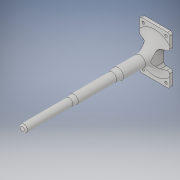
# Autodesk Inventor part: TapaInferiorConPata-v2
Saved by Autodesk Inventor 2019 (Build 230136000, 136)
## iProperties
Created: 2019-03-04
Part Number: TapaInferiorConPata-v2
Material: Generic
Document SubType Name: Modeling
Designer: Kenny
Density: 1 g/cm^3
Appearance: Default
Author: Kenny
Autodesk Inventor part; units mm, degrees
ref_plane "YZ Plane" through (0, 0, 0) normal (1, 0, 0) x (0, 1, 0)
ref_plane "XZ Plane" through (0, 0, 0) normal (0, 1, 0) x (-1, 0, 0)
ref_plane "XY Plane" through (0, 0, 0) normal (0, 0, 1) x (1, 0, 0)
sketch "Sketch1" plane through (0, 0, 0) normal (0, 0, 1) x (1, 0, 0)
  line L0 (41, 0) -> (41, 65.3) construction
  line L1 (0, 65.3) -> (0, 0) construction
  line L2 (41, 0) -> (41, 21)
  line L3 (0, 21) -> (0, 0)
  line L4 (41, 65.3) -> (41, 44.3)
  line L5 (0, 44.3) -> (0, 65.3)
  line L6 (29, 44.3) -> (29, 21)
  line L7 (12, 21) -> (12, 44.3)
  line L8 (41, 44.3) -> (29, 44.3)
  line L9 (12, 44.3) -> (0, 44.3)
  line L10 (41, 21) -> (29, 21)
  line L11 (12, 21) -> (0, 21)
  line L12 (41, 65.3) -> (30.5, 65.3) construction
  line L13 (10.5, 65.3) -> (0, 65.3) construction
  line L14 (0, 65.3) -> (10.5, 65.3)
  line L15 (30.5, 65.3) -> (41, 65.3)
  line L16 (0, 0) -> (10.5, 0) construction
  line L17 (30.5, 0) -> (41, 0) construction
  line L18 (0, 0) -> (10.5, 0)
  line L19 (30.5, 0) -> (41, 0)
  line L20 (10.5, 65.3) -> (30.5, 65.3)
  line L21 (10.5, 0) -> (30.5, 0)
  point P0 (5, 60.3)
  point P1 (36, 60.3)
  point P2 (5, 5)
  point P3 (36, 5)
  dimension "d0" = 41
  dimension "d1" = 65.3
  dimension "d2" = 21
  dimension "d3" = 21
  dimension "d4" = 12
  dimension "d9" = 5
  dimension "d11" = 5
  dimension "d12" = 41
  dimension "d13" = 41
  dimension "d14" = 12
  dimension "d19" = 5
  dimension "d20" = 5
  constraints: 44 end point, 17 parallel, 6 horizontal, 6 perpendicular, 2 horizontal alignment, 2 vertical alignment
  measures "d0" distance of L1.start L0.end
  measures "d1" distance of L0.end L0.start
  measures "d2" distance of L2.end L2.start
  measures "d3" distance of L4.start L4.end
  measures "d4" distance between parallel lines of L0 L6
  measures "d9" distance from line of L1 point (5, 60.3)
  measures "d11" distance from line of L0 point (36, 60.3)
  measures "d12" distance between parallel lines of L1 L2
  measures "d13" distance between parallel lines of L1 L4
  measures "d14" distance between parallel lines of L3 L7
  measures "d19" distance from line of L13 point (5, 60.3)
  measures "d20" distance from line of L16 point (5, 5)
extrude "Extrusion3" add sketch "Sketch1" along normal blind 4
sketch "Sketch5" plane through (0, 0, 0) normal (0, 0, 1) x (1, 0, 0)
  line L0 (41, 0) -> (41, 65.3) construction
  line L1 (0, 65.3) -> (0, 0) construction
  line L2 (41, 0) -> (41, 21)
  line L3 (0, 21) -> (0, 0)
  line L4 (41, 65.3) -> (41, 44.3)
  line L5 (0, 44.3) -> (0, 65.3)
  line L6 (29, 44.3) -> (29, 21)
  line L7 (12, 21) -> (12, 44.3)
  line L8 (41, 44.3) -> (29, 44.3)
  line L9 (12, 44.3) -> (0, 44.3)
  line L10 (41, 21) -> (29, 21)
  line L11 (12, 21) -> (0, 21)
  line L12 (30.5, 65.3) -> (30.5, 55.3)
  line L13 (30.5, 55.3) -> (10.5, 55.3)
  line L14 (10.5, 55.3) -> (10.5, 65.3)
  line L15 (41, 65.3) -> (30.5, 65.3) construction
  line L16 (10.5, 65.3) -> (0, 65.3) construction
  line L17 (0, 65.3) -> (10.5, 65.3)
  line L18 (30.5, 65.3) -> (41, 65.3)
  line L19 (10.5, 0) -> (10.5, 10)
  line L20 (10.5, 10) -> (30.5, 10)
  line L21 (30.5, 10) -> (30.5, 0)
  line L22 (0, 0) -> (10.5, 0) construction
  line L23 (30.5, 0) -> (41, 0) construction
  line L24 (0, 0) -> (10.5, 0)
  line L25 (30.5, 0) -> (41, 0)
  point P0 (5, 60.3)
  point P1 (36, 60.3)
  point P2 (5, 5)
  point P3 (36, 5)
  dimension "d53" = 41
  dimension "d54" = 65.3
  dimension "d55" = 21
  dimension "d56" = 21
  dimension "d57" = 12
  dimension "d58" = 5
  dimension "d59" = 5
  dimension "d60" = 41
  dimension "d61" = 41
  dimension "d62" = 12
  dimension "d63" = 10.5
  dimension "d64" = 10.5
  dimension "d65" = 5
  dimension "d66" = 5
  constraints: 52 end point, 18 parallel, 6 horizontal, 6 perpendicular, 2 horizontal alignment, 2 vertical alignment
  measures "d53" distance of L1.start L0.end
  measures "d54" distance of L0.end L0.start
  measures "d55" distance of L2.end L2.start
  measures "d56" distance of L4.start L4.end
  measures "d57" distance between parallel lines of L0 L6
  measures "d58" distance from line of L1 point (5, 60.3)
  measures "d59" distance from line of L0 point (36, 60.3)
  measures "d60" distance between parallel lines of L1 L2
  measures "d61" distance between parallel lines of L1 L4
  measures "d62" distance between parallel lines of L3 L7
  measures "d63" distance between parallel lines of L5 L14
  measures "d64" distance between parallel lines of L0 L12
  measures "d65" distance from line of L16 point (5, 60.3)
  measures "d66" distance from line of L22 point (5, 5)
hole "Hole2" at (5, 60.3, 0) at (36, 60.3, 0) at (5, 5, 0) at (36, 5, 0) direction (0, 0, 1) diameter 3.6 end through all
fillet "Fillet2" radius 3 12 edges at (0, 65.3, 2) (41, 65.3, 2) (41, 44.3, 2) (29, 44.3, 2) (29, 21, 2) (41, 21, 2) (41, 0, 2) (0, 0, 2) (0, 44.3, 2) (12, 44.3, 2) (12, 21, 2) (0, 21, 2)
sketch "Sketch6" plane through (0, 0, 4) normal (0, 0, 1) x (1, 0, 0)
  line L0 (12, 21) -> (12, 44.3) projected
  line L1 (29, 44.3) -> (29, 21) projected
  circle A0 centre (20.5, 32.65) radius 7.5
  line L2 (41, 65.3) -> (0, 65.3) projected
  point P0 (0, 0)
  dimension "d76" = 15
  dimension "d79" = 8.5
  dimension "d80" = 32.65
  constraints: 1 centre point
  measures "d76" diameter of A0
  measures "d79" distance from line of L1 A0.centre
  measures "d80" distance from line of L2 A0.centre
extrude "Extrusion4" add sketch "Sketch6" along normal blind 50
sketch "Sketch7" plane through (20.5, 32.65, 54) normal (0, 0, 1) x (1, 0, 0)
  circle A0 centre (0, 0) radius 6
  point P0 (-20.5, -32.65)
  dimension "d83" = 12
  constraints: 1 centre point
  measures "d83" diameter of A0
extrude "Extrusion5" add sketch "Sketch7" along normal blind 60
sketch "Sketch8" plane through (20.5, 32.65, 114) normal (0, 0, 1) x (1, 0, 0)
  circle A0 centre (0, 0) radius 5
  point P0 (-20.5, -32.65)
  dimension "d86" = 10
  constraints: 1 centre point
  measures "d86" diameter of A0
extrude "Extrusion6" add sketch "Sketch8" along normal blind 70
fillet "Fillet5" radius 2 1 edges at (15.5, 32.65, 184)
fillet "Fillet6" radius 20 2 edges at (15.5, 32.65, 114) (14.5, 32.65, 54)
fillet "Fillet7" radius 20 1 edges at (13, 32.65, 4)
body "Solid2"
